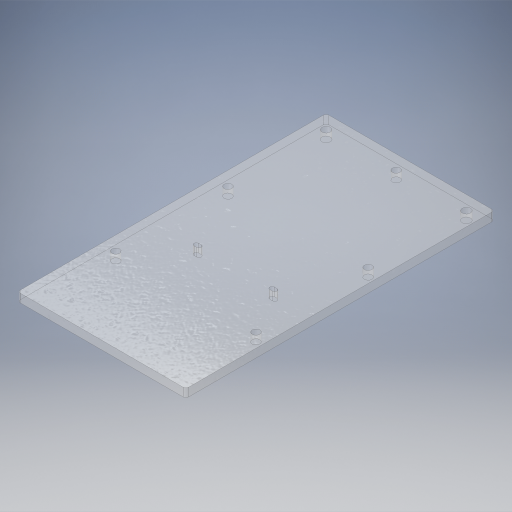
# Autodesk Inventor part: BT005_trajan20_21
Saved by Autodesk Inventor 2023 (Build 270158000, 158)
## iProperties
Company: HTBLA Kaindorf
RuleStatus: InUse
Created: 2022-08-07
Part Number: BT005_trajan20_21
Project: Zeichenmaschine_v2
Material: Acryl
Description: getriebemotor platte unten
Document SubType Name: Modeling
Designer: trajan20
Density: 1.188 g/cm^3
Appearance: Transparent - farblos
Mass: 186.699 g
Surface Area: 573.573 cm^2
Volume: 157.154 cm^3
AfterDocNew0: iProperties-Editor_aufrufen
Author: jan
Keywords: 2021
Autodesk Inventor part; units mm, degrees
ref_plane "YZ Plane" through (0, 0, 0) normal (1, 0, 0) x (0, 1, 0)
sketch "Skizze3" plane through (0, 0, 0) normal (0, 0, 1) x (1, 0, 0)
  line L0 (0, 0) -> (-220, 0)
  line L1 (-220, 0) -> (-220, 120)
  line L2 (-220, 120) -> (0, 120)
  line L3 (0, 120) -> (0, 0)
  point P0 (-210, 60)
  point P1 (-140, 10)
  point P2 (-140, 110)
  point P3 (-220, 60)
  point P4 (-60, 10)
  point P5 (-60, 110)
  point P6 (-210, 10)
  point P7 (-210, 110)
  dimension "d4" = 120
  dimension "d5" = 220
  dimension "d31" = 10
  dimension "d32" = 10
  dimension "d33" = 10
  dimension "d34" = 80
  dimension "d42" = 60
  constraints: 8 end point, 5 horizontal alignment, 4 vertical alignment, 2 parallel, 1 horizontal, 1 midpoint, 1 perpendicular
  measures "d4" distance between parallel lines of L0 L2
  measures "d5" distance between parallel lines of L1 L3
  measures "d31" distance from line of L1 point (-210, 60)
  measures "d32" distance from line of point (-140, 110) L2
  measures "d33" distance from line of L0 point (-140, 10)
  measures "d34" distance from line of L1 point (-140, 10)
  measures "d42" distance from line of L3 point (-60, 110)
extrude "Extrusion3" add sketch "Skizze3" along normal blind 6
ref_plane "Arbeitsebene1" through (-110, 120, 6) normal (-1, 0, 0) x (0, -1, 0)
ref_plane "Arbeitsebene2" through (-220, 60, 6) normal (0, -1, 0) x (1, 0, 0)
fillet "Rundung2" radius 2 4 edges at (0, 0, 3) (0, 120, 3) (-220, 120, 3) (-220, 0, 3)
derived "BT000_trajan20_22_Zeichenmaschine_neu_Masterskizze.ipt"
hole "Bohrung2" at (-210, 60, 0) at (-140, 10, 0) at (-140, 110, 0) at (-60, 110, 0) at (-60, 10, 0) direction (0, 0, 1) diameter 5.5 end through all
hole "Bohrung3" at (-210, 10, 0) at (-210, 110, 0) direction (0, 0, 1) diameter 6 end through all
derived "BT102_trajan20_21_Zeichenmaschine_v2_Platte Getriebemotor.ip"
sketch "Skizze6" plane through (0, 0, -5) normal (0, 0, -1) x (-1, 0, 0)
  circle A0 centre (60, 110) radius 2.75
  circle A1 centre (140, 10) radius 2.75
  circle A2 centre (60, 10) radius 2.75
  circle A3 centre (140, 110) radius 2.75
  circle A4 centre (210, 60) radius 2.75
  arc A5 (0, 2) -> (2, 0) centre (2, 2) ccw
  line L0 (2, 0) -> (218, 0)
  arc A6 (218, 0) -> (220, 2) centre (218, 2) ccw
  line L1 (220, 2) -> (220, 118)
  arc A7 (220, 118) -> (218, 120) centre (218, 118) ccw
  line L2 (218, 120) -> (2, 120)
  arc A8 (2, 120) -> (0, 118) centre (2, 118) ccw
  line L3 (0, 118) -> (0, 2)
  circle A9 centre (179.05, 69.25) radius 3.775
  line L4 (138.8, 76) -> (184.8, 76)
  line L5 (184.8, 76) -> (184.8, 44)
  circle A10 centre (179.05, 50.75) radius 3.775
  circle A11 centre (179.05, 50.75) radius 1.55
  line L6 (184.8, 44) -> (138.8, 44)
  line L7 (138.8, 44) -> (138.8, 76)
  line L8 (153.75, 65) -> (153.75, 55)
  arc A12 (159.95, 65) -> (153.75, 65) centre (156.85, 65) ccw
  line L9 (159.95, 55) -> (159.95, 65)
  arc A13 (153.75, 55) -> (159.95, 55) centre (156.85, 55) ccw
  circle A14 centre (145.55, 50.75) radius 3.775
  circle A15 centre (145.55, 50.75) radius 1.55
  circle A16 centre (145.55, 69.25) radius 3.775
  circle A17 centre (145.55, 69.25) radius 1.55
  circle A18 centre (170, 60) radius 6.675
  circle A19 centre (170, 60) radius 3.1
  circle A20 centre (179.05, 69.25) radius 1.55
  line L10 (123.8, 84) -> (192.8, 84)
  line L11 (192.8, 84) -> (192.8, 36)
  line L12 (192.8, 36) -> (123.8, 36)
  line L13 (123.8, 36) -> (123.8, 84)
  line L14 (138.8, 62.6) -> (95.8, 62.6)
  line L15 (138.8, 57.6) -> (95.8, 57.6)
  line L16 (95.8, 67.6) -> (138.8, 67.6)
  line L17 (138.8, 67.6) -> (138.8, 57.6)
  line L18 (138.8, 57.6) -> (95.8, 67.6)
  line L19 (95.8, 57.6) -> (138.8, 67.6)
  line L20 (89.7, 99.6) -> (95.8, 99.6)
  line L21 (89.7, 25.6) -> (89.7, 99.6)
  line L22 (89.7, 83.85) -> (39.7, 83.85)
  line L23 (39.7, 41.35) -> (89.7, 41.35)
  line L24 (95.8, 99.6) -> (95.8, 25.6)
  line L25 (95.8, 25.6) -> (89.7, 25.6)
  line L26 (39.7, 41.35) -> (39.7, 83.85)
  line L27 (103.8, 90.6) -> (103.8, 88.6)
  line L28 (102.2, 90.6) -> (102.2, 88.6)
  line L29 (105.4, 88.6) -> (105.4, 90.6)
  arc A21 (105.4, 90.6) -> (102.2, 90.6) centre (103.8, 90.6) ccw
  arc A22 (102.2, 88.6) -> (105.4, 88.6) centre (103.8, 88.6) ccw
  line L30 (103.8, 36.6) -> (103.8, 34.6)
  line L31 (102.2, 36.6) -> (102.2, 34.6)
  line L32 (105.4, 34.6) -> (105.4, 36.6)
  arc A23 (105.4, 36.6) -> (102.2, 36.6) centre (103.8, 36.6) ccw
  arc A24 (102.2, 34.6) -> (105.4, 34.6) centre (103.8, 34.6) ccw
  point P0 (0, 0)
  point P1 (138.8, 60)
  point P2 (123.8, 60)
  point P3 (117.3, 62.6)
  point P4 (92.3, 62.6)
  point P5 (95.8, 62.6)
  point P6 (89.7, 62.6)
  point P7 (39.7, 62.6)
  point P8 (103.8, 89.6)
  point P9 (103.8, 35.6)
  point P10 (92.75, 25.6)
sketch "Skizze5" plane through (0, 0, 6) normal (0, 0, 1) x (1, 0, 0)
  line L0 (-95.8, 99.6) -> (-95.8, 25.6) projected
  line L1 (-103.8, 35.6) -> (-92.8, 35.6) construction
  line L2 (-103.8, 89.6) -> (-92.8, 89.6) construction
  line L3 (-92.8, 34.6) -> (-92.8, 36.6) construction
  line L4 (-91.2, 34.6) -> (-91.2, 36.6)
  line L5 (-94.4, 36.6) -> (-94.4, 34.6)
  arc A0 (-94.4, 34.6) -> (-91.2, 34.6) centre (-92.8, 34.6) ccw
  arc A1 (-91.2, 36.6) -> (-94.4, 36.6) centre (-92.8, 36.6) ccw
  line L6 (-92.8, 88.6) -> (-92.8, 90.6) construction
  line L7 (-91.2, 88.6) -> (-91.2, 90.6)
  line L8 (-94.4, 90.6) -> (-94.4, 88.6)
  arc A2 (-94.4, 88.6) -> (-91.2, 88.6) centre (-92.8, 88.6) ccw
  arc A3 (-91.2, 90.6) -> (-94.4, 90.6) centre (-92.8, 90.6) ccw
  line L9 (-89.7, 25.6) -> (-89.7, 99.6) projected
  line L10 (-102.2, 36.6) -> (-102.2, 34.6) projected
  arc A4 (-105.4, 34.6) -> (-102.2, 34.6) centre (-103.8, 34.6) ccw projected
  line L11 (-105.4, 34.6) -> (-105.4, 36.6) projected
  arc A5 (-102.2, 36.6) -> (-105.4, 36.6) centre (-103.8, 36.6) ccw projected
  line L12 (-103.8, 36.6) -> (-103.8, 34.6) projected
  line L13 (-103.8, 90.6) -> (-103.8, 88.6) projected
  point P0 (0, 0)
  dimension "d51" = 3
  dimension "d52" = 3
  dimension "d53" = 1.6
  dimension "d54" = 2
  dimension "d55" = 2
  dimension "d56" = 1.6
  dimension "d59" = 2
  dimension "d60" = 2
  constraints: 20 end point, 8 point on circle, 8 tangent, 4 centre point, 2 horizontal, 2 midpoint, 2 parallel, 2 vertical
  measures "d51" distance from line of L2.end L0
  measures "d52" distance from line of L1.end L0
  measures "d53" radius of A1
  measures "d54" distance of L3.start L3.end
  measures "d55" distance of L6.start L6.end
  measures "d56" radius of A3
  measures "d59" distance of L13.start L13.end
  measures "d60" distance of L12.start L12.end
extrude "Extrusion5" cut sketch "Skizze5" against normal blind 10 contours A0 L5 A1 L4 | A2 L8 A3 L7
equation "\"d4\" = Basis_Zubau_Breite_Profillänge + 4 * AluProfil_Abstand"
equation "\"d5\" = Basis_Zubau_Länge_Profillänge + 2 * AluProfil_Abstand"
equation "\"d31\" = AluProfil_Abstand"
equation "\"d32\" = AluProfil_Abstand"
equation "\"d33\" = AluProfil_Abstand"
equation "\"d54\" = d60"
equation "\"d55\" = d59"
equation "\"Basis_Zubau_Breite_Profillänge\" = 80"
equation "\"AluProfil_Abstand\" = 10"
equation "\"Basis_Zubau_Länge_Profillänge\" = 200"
